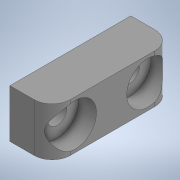
# Autodesk Inventor part: beltClamp
Saved by Autodesk Inventor 2022 (Build 260153000, 153)
## iProperties
Created: 2021-11-29
Part Number: beltClamp
Material: Polycarbonate, Clear
Document SubType Name: Modeling
Designer: alexr
Density: 1.2 g/cm^3
Appearance: Polycarbonate - Clear
Author: alexr
Autodesk Inventor part; units mm, degrees
ref_plane "YZ Plane" through (0, 0, 0) normal (1, 0, 0) x (0, 1, 0)
ref_plane "XZ Plane" through (0, 0, 0) normal (0, 1, 0) x (-1, 0, 0)
ref_plane "XY Plane" through (0, 0, 0) normal (0, 0, 1) x (1, 0, 0)
sketch "Sketch1" plane through (0, 0, 0) normal (1, 0, 0) x (0, 1, 0)
  circle A0 centre (0, 7.0915) radius 1.6
  circle A1 centre (0, -4.9085) radius 1.6
  line L0 (-4, 10.9179) -> (4, 10.9179)
  line L1 (4, 10.9179) -> (4, -9.0821)
  line L2 (4, -9.0821) -> (-4, -9.0821)
  line L3 (-4, -9.0821) -> (-4, 10.9179)
  line L4 (-4, 10.9179) -> (4, -9.0821) construction
  line L5 (4, 10.9179) -> (-4, -9.0821) construction
  point P0 (0, 0.9179)
  dimension "d0" = 3.2
  dimension "d1" = 3.2
  dimension "d2" = 12
  dimension "d6" = 8
  dimension "d7" = 20
  constraints: 12 end point, 2 centre point, 2 midpoint, 2 parallel, 1 horizontal, 1 perpendicular
  measures "d0" diameter of A0
  measures "d1" diameter of A1
  measures "d2" distance of A1.centre A0.centre
  measures "d6" distance of L1.end L2.end
  measures "d7" distance of L0.end L1.end
extrude "Extrusion1" add sketch "Sketch1" along normal blind 4
sketch "Sketch2" plane through (4, 0, 0) normal (1, 0, 0) x (0, 0, -1)
  circle A0 centre (-7.0915, 0) radius 1.6 projected
  circle A1 centre (-7.0915, 0) radius 3.5
  circle A2 centre (4.9085, 0) radius 1.6 projected
  circle A3 centre (4.9085, 0) radius 3.5
  line L0 (9.0821, -4) -> (9.0821, 4) projected
  line L1 (9.0821, 4) -> (-10.9179, 4) projected
  line L2 (-10.9179, 4) -> (-10.9179, -4) projected
  line L3 (-10.9179, -4) -> (9.0821, -4) projected
  circle A4 centre (4.9085, 0) radius 1.6 projected
  circle A5 centre (-7.0915, 0) radius 1.6 projected
  point P0 (0, 0)
  dimension "d10" = 7
  dimension "d11" = 7
  constraints: 2 centre point, 2 coincident
  measures "d10" diameter of A1
  measures "d11" diameter of A3
extrude "Extrusion2" add sketch "Sketch2" along normal blind 3 contours L3 L2 L1 L0
fillet "Fillet1" radius 3 2 edges at (7, 0, 10.9179) (7, 0, -9.0821)
sketch "Sketch3" plane through (0, 0, 0) normal (-1, 0, 0) x (0, 0, 1)
  line L0 (4.5915, 2.5) -> (-2.4085, 2.5)
  line L1 (-2.4085, 2.5) -> (-2.4085, 3.5)
  line L2 (-2.4085, 3.5) -> (4.5915, 3.5)
  line L3 (4.5915, 3.5) -> (4.5915, 2.5)
  line L4 (4.5915, 2.5) -> (-2.4085, 3.5) construction
  line L5 (-2.4085, 2.5) -> (4.5915, 3.5) construction
  circle A0 centre (-4.9085, 0) radius 1.6 projected
  circle A1 centre (7.0915, 0) radius 1.6 projected
  line L6 (-9.0821, 4) -> (10.9179, 4) projected
  line L7 (-2.4085, 0.5) -> (-2.4085, 1.5)
  line L8 (4.5915, 0.5) -> (-2.4085, 0.5)
  line L9 (-2.4085, 1.5) -> (4.5915, 1.5)
  line L10 (4.5915, 1.5) -> (4.5915, 0.5)
  line L11 (-2.4085, -1.5) -> (-2.4085, -0.5)
  line L12 (4.5915, -1.5) -> (-2.4085, -1.5)
  line L13 (-2.4085, -0.5) -> (4.5915, -0.5)
  line L14 (4.5915, -0.5) -> (4.5915, -1.5)
  line L15 (-2.4085, -3.5) -> (-2.4085, -2.5)
  line L16 (4.5915, -3.5) -> (-2.4085, -3.5)
  line L17 (-2.4085, -2.5) -> (4.5915, -2.5)
  line L18 (4.5915, -2.5) -> (4.5915, -3.5)
  point P0 (0, 0)
  point P1 (1.0915, 3)
  dimension "d15" = 7
  dimension "d16" = 12
  dimension "d17" = 6
  dimension "d18" = 1
  dimension "d19" = 0.5
  dimension "d22" = 2
  constraints: 36 end point, 2 midpoint, 2 parallel, 1 collinear, 1 horizontal, 1 perpendicular, 1 vertical, 23 other
  measures "d15" distance of L1.end L2.end
  measures "d16" distance of A0.centre A1.centre
  measures "d17" horizontal distance of A0.centre point (1.091, 3)
  measures "d18" distance of L2.end L0.start
  measures "d19" distance between parallel lines of L6 L2
  measures "d22" distance of L0.end L7.start
extrude "Extrusion3" add sketch "Sketch3" along normal blind 0.5 contours L0 L1 L2 L3 | L7 L9 L10 L8 | L11 L13 L14 L12 | L15 L17 L18 L16
fillet "Fillet2" radius 0.25 16 edges at (-0.5, -2.5, 1.0915) (0, -2.5, 1.0915) (-0.5, -1.5, 1.0915) (-0.5, -0.5, 1.0915) (-0.5, 0.5, 1.0915) (-0.5, 1.5, 1.0915) (-0.5, 2.5, 1.0915) (-0.5, 3.5, 1.0915) (0, 3.5, 1.0915) (0, 2.5, 1.0915) (0, 1.5, 1.0915) (0, 0.5, 1.0915) (0, -0.5, 1.0915) (0, -1.5, 1.0915) (0, -3.5, 1.0915) (-0.5, -3.5, 1.0915)
equation "\"d10\" = d11"
equation "\"d17\" = 0.5 * d16"
body "Solid1"
